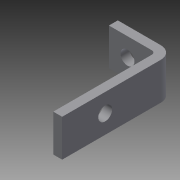
# Autodesk Inventor part: PistonFrontHinge
Saved by Autodesk Inventor 2013 (Build 170138000, 138)
## iProperties
Created: 2013-02-07
Part Number: PistonFrontHinge
Material: Generic
Document SubType Name: Sheet Metal
Designer: motoennies
Density: 1 g/cm^3
Sheet Metal Rule: Default
Author: motoennies
Autodesk Inventor part; units mm, degrees
ref_plane "YZ Plane" through (0, 0, 0) normal (1, 0, 0) x (0, 1, 0)
ref_plane "XZ Plane" through (0, 0, 0) normal (0, 1, 0) x (-1, 0, 0)
ref_plane "XY Plane" through (0, 0, 0) normal (0, 0, 1) x (1, 0, 0)
sketch "Sketch1" plane through (0, 0, 0) normal (0, 0, 1) x (1, 0, 0)
  circle A0 centre (0, 0) radius 2.3876
  line L0 (12.7, 0) -> (12.7, 6.35)
  line L1 (12.7, -6.35) -> (12.7, 0)
  line L2 (-6.35, -6.35) -> (-6.35, 6.35)
  line L3 (-6.35, 6.35) -> (12.7, 6.35)
  line L4 (-6.35, -6.35) -> (12.7, -6.35)
  dimension "d0" = 4.7752
  dimension "d1" = 6.35
  dimension "d4" = 12.7
  dimension "d22" = 19.05
  dimension "d23" = 12.7
  measures "d0" diameter of A0
  measures "d1" distance of L0.start L0.end
  measures "d4" distance from line of A0.centre L0
  measures "d22" distance between parallel lines of L1 L2
  measures "d23" distance between parallel lines of L4 L3
extrude "Plate1" add sketch "Sketch1" along normal blind 3.048
sketch "Sketch2" plane through (9.652, 6.35, 0) normal (1, 0, 0) x (0, 1, 0)
  line L0 (-12.7, 0) -> (0, 0)
  line L1 (0, 0) -> (0, 38.1)
  line L2 (0, 38.1) -> (-12.7, 38.1)
  line L3 (-12.7, 38.1) -> (-12.7, 0)
  constraints: 6 end point, 1 horizontal, 1 perpendicular, 1 vertical
edge flange "Flange1" height 38.1 angle 90 thickness 3.048 bend radius 1.27 thickness toward (1, 0, 0) relief tear relief width 3.048 relief depth 1.524 edges at (12.7, 3.175, 3.048) wall of the first edge with corners at (9.652, -6.35, 0) (9.652, 6.35, 0) (9.652, 6.35, 38.1) (9.652, -6.35, 38.1)
bend "Bend1"
corner "Corner1"
sketch "Sketch3" plane through (12.7, -6.35, 38.1) normal (1, 0, 0) x (0, 0, -1)
  circle A0 centre (14.732, 6.35) radius 2.3812
  line L0 (33.782, 0) -> (33.782, 12.7) projected
  line L1 (33.782, 0) -> (0, 0) projected
  point P0 (38.1, 6.35)
  dimension "d17" = 4.7625
  dimension "d20" = 6.35
  dimension "d21" = 19.05
  constraints: 1 centre point
  measures "d17" diameter of A0
  measures "d20" distance from line of L1 A0.centre
  measures "d21" distance from line of L0 A0.centre
extrude "Extrusion1" cut sketch "Sketch3" against normal blind 25.4
equation "\"d7\" = BendReliefWidth"
equation "\"d8\" = BendReliefDepth"
equation "\"d9\" = MinimumRemnant"
equation "\"d10\" = BendRadius"
equation "\"d14\" = CornerReliefSize"
equation "\"d15\" = GapSize"
equation "\"d16\" = JacobiRadiusSize"
equation "\"BendRadius\" = Thickness"
equation "\"BendReliefWidth\" = Thickness"
equation "\"BendReliefDepth\" = 0.5 * Thickness"
equation "\"CornerReliefSize\" = 4 * Thickness"
equation "\"MinimumRemnant\" = 2 * Thickness"
equation "\"TransitionRadius\" = BendRadius"
equation "\"JacobiRadiusSize\" = BendRadius"
equation "\"GapSize\" = Thickness"
equation "\"d6\" = BendRadius"
equation "\"Thickness\" = 3.048"
body "Solid1"
